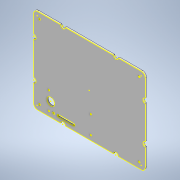
# Autodesk Inventor part: AcrylicCover
Saved by Autodesk Inventor 2022 (Build 260153000, 153)
## iProperties
Created: 2021-11-11
Part Number: AcrylicCover
Material: Generic
Document SubType Name: Modeling
Designer: Viktor
Density: 1 g/cm^3
Appearance: Default
Author: Viktor
Autodesk Inventor part; units mm, degrees
ref_plane "YZ Plane" through (0, 0, 0) normal (1, 0, 0) x (0, 1, 0)
ref_plane "XZ Plane" through (0, 0, 0) normal (0, 1, 0) x (-1, 0, 0)
ref_plane "XY Plane" through (0, 0, 0) normal (0, 0, 1) x (1, 0, 0)
sketch "Sketch1" plane through (0, 0, 0) normal (0, 0, 1) x (1, 0, 0)
  line L0 (-117, -89.5) -> (117, -89.5)
  line L1 (117, -89.5) -> (117, 89.5)
  line L2 (117, 89.5) -> (-117, 89.5)
  line L3 (-117, 89.5) -> (-117, -89.5)
  line L4 (-117, -89.5) -> (117, 89.5) construction
  line L5 (117, -89.5) -> (-117, 89.5) construction
  point P0 (0, 0)
  dimension "d0" = 234
  dimension "d1" = 179
  constraints: 12 end point, 2 midpoint, 2 parallel, 1 horizontal, 1 perpendicular
  measures "d0" distance between parallel lines of L1 L3
  measures "d1" distance between parallel lines of L0 L2
extrude "Extrusion1" add sketch "Sketch1" along normal blind 3
fillet "Fillet1" radius 8 4 edges at (117, -89.5, 1.5) (-117, -89.5, 1.5) (-117, 89.5, 1.5) (117, 89.5, 1.5)
sketch "Sketch2" plane through (0, 0, 3) normal (0, 0, 1) x (1, 0, 0)
  line L0 (-109, -89.5) -> (109, -89.5) construction
  arc A0 (-117, -81.5) -> (-109, -89.5) centre (-109, -81.5) ccw projected
  line L1 (-117, 81.5) -> (-117, -81.5) projected
  arc A1 (-109, 89.5) -> (-117, 81.5) centre (-109, 81.5) ccw projected
  line L2 (109, 89.5) -> (-109, 89.5) projected
  arc A2 (117, 81.5) -> (109, 89.5) centre (109, 81.5) ccw projected
  line L3 (117, -81.5) -> (117, 81.5) construction
  arc A3 (109, -89.5) -> (117, -81.5) centre (109, -81.5) ccw construction
  line L4 (-109, -89.5) -> (109, -89.5) projected
  circle A4 centre (55.5, -89.5) radius 5
  line L5 (117, -81.5) -> (117, 81.5) projected
  circle A5 centre (117, -39.5) radius 5
  line L6 (-170.275, 0) -> (170.275, 0) projected
  line L7 (0, 131.775) -> (0, -131.775) projected
  arc A6 (-117, -81.5) -> (-109, -89.5) centre (-109, -81.5) ccw construction
  circle A7 centre (-55.5, -89.5) radius 5
  circle A8 centre (-117, -39.5) radius 5
  line L8 (-109, 89.5) -> (109, 89.5) construction
  arc A9 (-109, 89.5) -> (-117, 81.5) centre (-109, 81.5) ccw
  arc A10 (117, 81.5) -> (109, 89.5) centre (109, 81.5) ccw construction
  line L9 (-109, 89.5) -> (109, 89.5)
  circle A11 centre (55.5, 89.5) radius 5
  circle A12 centre (117, 39.5) radius 5
  circle A13 centre (-117, 39.5) radius 5
  arc A14 (-109, 89.5) -> (-117, 81.5) centre (-109, 81.5) ccw construction
  circle A15 centre (-55.5, 89.5) radius 5
  point P0 (0, 0)
  point P1 (-50.5, -89.5)
  point P2 (-60.5, -89.5)
  point P3 (-117, -34.5)
  point P4 (-117, -44.5)
  point P5 (-117, 44.5)
  point P6 (-117, 34.5)
  point P7 (-60.5, 89.5)
  point P8 (-50.5, 89.5)
  point P9 (50.5, 89.5)
  point P10 (60.5, 89.5)
  point P11 (117, 44.5)
  point P12 (117, 34.5)
  point P13 (117, -34.5)
  point P14 (117, -44.5)
  point P15 (60.5, -89.5)
  point P16 (50.5, -89.5)
  dimension "d5" = 10
  dimension "d6" = 10
  dimension "d7" = 61.5
  dimension "d8" = 50
  constraints: 12 centre point, 10 symmetric about line, 8 point on circle, 4 end point, 3 point on line, 10 other
  measures "d5" diameter of A4
  measures "d6" diameter of A5
  measures "d7" distance from line of L3 A4.centre
  measures "d8" distance from line of L0 A5.centre
extrude "Extrusion2" cut sketch "Sketch2" against normal through all contours L5 A5 | A4 L4 | L1 A8 | A7 L4 | L1 A13 | A12 L5 | L2 A11 | A15 L2 picked at (116.6011, -41.1182) picked at (57.1182, -89.1011) picked at (-115.906, -37.9566) picked at (-53.8818, -89.1011) picked at (-115.906, 41.0434) picked at (115.4959, 40.7959) picked at (57.0242, 88.3266) picked at (-53.9758, 88.3266)
sketch "Sketch3" plane through (0, 0, 3) normal (0, 0, 1) x (1, 0, 0)
  circle A0 centre (104.5, -77.5) radius 1.75
  line L0 (117, -34.5) -> (117, 34.5) projected
  line L1 (60.5, -89.5) -> (109, -89.5) construction
  line L2 (0, 127.7397) -> (0, -127.7397) projected
  line L3 (-166.2397, 0) -> (166.2397, 0) projected
  circle A1 centre (-104.5, -77.5) radius 1.75
  circle A2 centre (104.5, 77.5) radius 1.75
  line L4 (60.5, 89.5) -> (109, 89.5) construction
  circle A3 centre (-104.5, 77.5) radius 1.75
  point P0 (0, 0)
  point P1 (-109, -89.5)
  point P2 (-109, 89.5)
  dimension "d11" = 3.5
  dimension "d33" = 209
  dimension "d34" = 155
  constraints: 7 symmetric about line, 4 centre point, 2 end point, 3 other
  measures "d11" diameter of A0
  measures "d33" distance of A1.centre A0.centre
  measures "d34" distance of A3.centre A1.centre
extrude "Extrusion3" cut sketch "Sketch3" against normal blind 10
sketch "Sketch4" plane through (0, 0, 3) normal (0, 0, 1) x (1, 0, 0)
  circle A0 centre (-81, -60.5) radius 8
  circle A1 centre (-75, -78.5) radius 2
  line L0 (-33, -78.5) -> (-65, -78.5) construction
  line L1 (-33, -76) -> (-65, -76)
  line L2 (-65, -81) -> (-33, -81)
  arc A2 (-33, -81) -> (-33, -76) centre (-33, -78.5) ccw
  arc A3 (-65, -76) -> (-65, -81) centre (-65, -78.5) ccw
  circle A4 centre (-85, -79.5) radius 1.5
  line L3 (-12.5, -60.5) -> (-95.5, -60.5) construction
  line L4 (-41, -83.5) -> (-41, -33.5) construction
  circle A5 centre (3, -79.5) radius 1.5
  circle A6 centre (-85, -41.5) radius 1.5
  circle A7 centre (3, -41.5) radius 1.5
  line L5 (-109, -89.5) -> (-60.5, -89.5) projected
  line L6 (-117, -44.5) -> (-117, -81.5) projected
  point P0 (0, 0)
  point P1 (-49, -78.5)
  dimension "d16" = 2.5
  dimension "d17" = 16
  dimension "d18" = 4
  dimension "d19" = 10
  dimension "d20" = 32
  dimension "d21" = 6
  dimension "d22" = 18
  dimension "d23" = 34
  dimension "d24" = 18
  dimension "d25" = 44
  dimension "d26" = 19
  dimension "d27" = 3
  dimension "d28" = 10
  dimension "d29" = 32
  dimension "d30" = 0
  constraints: 12 end point, 8 centre point, 4 point on circle, 4 tangent, 3 symmetric about line, 2 horizontal, 1 midpoint, 1 parallel, 1 vertical, 3 other
  measures "d16" radius of A3
  measures "d17" diameter of A0
  measures "d18" diameter of A1
  measures "d19" distance of L0.end A1.centre
  measures "d20" distance of L0.end L0.start
  measures "d21" horizontal distance of A0.centre A1.centre
  measures "d22" vertical distance of A1.centre A0.centre
  measures "d23" distance from line of L4 A1.centre
  measures "d24" distance from line of A1.centre L3
  measures "d25" distance from line of L4 A4.centre
  measures "d26" distance from line of L3 A4.centre
  measures "d27" diameter of A4
  measures "d28" distance from line of L5 A4.centre
  measures "d29" distance from line of L6 A4.centre
  measures "d30" vertical distance of A1.centre point (-49, -78.5)
extrude "Extrusion4" cut sketch "Sketch4" against normal through all
sketch "Sketch5" plane through (0, 0, 3) normal (0, 0, 1) x (1, 0, 0)
  circle A0 centre (-81, -60.5) radius 8 projected
  line L0 (-33, -81) -> (-65, -81) projected
  arc A1 (-65, -76) -> (-65, -81) centre (-65, -78.5) ccw projected
  line L1 (-65, -76) -> (-33, -76) projected
  arc A2 (-33, -81) -> (-33, -76) centre (-33, -78.5) ccw projected
  circle A3 centre (-85, -41.5) radius 1.5 projected
  circle A4 centre (3, -41.5) radius 1.5 projected
  circle A5 centre (-75, -78.5) radius 2 projected
  circle A6 centre (-85, -79.5) radius 1.5 projected
  circle A7 centre (3, -79.5) radius 1.5 projected
  circle A8 centre (-104.5, 77.5) radius 1.75 projected
  circle A9 centre (-104.5, -77.5) radius 1.75 projected
  circle A10 centre (104.5, 77.5) radius 1.75 projected
  circle A11 centre (104.5, -77.5) radius 1.75 projected
  arc A12 (117, 44.5) -> (117, 34.5) centre (117, 39.5) ccw projected
  line L2 (117, 44.5) -> (117, 81.5) projected
  arc A13 (117, 81.5) -> (109, 89.5) centre (109, 81.5) ccw projected
  line L3 (109, 89.5) -> (60.5, 89.5) projected
  arc A14 (50.5, 89.5) -> (60.5, 89.5) centre (55.5, 89.5) ccw projected
  line L4 (50.5, 89.5) -> (-50.5, 89.5) projected
  arc A15 (-60.5, 89.5) -> (-50.5, 89.5) centre (-55.5, 89.5) ccw projected
  line L5 (-60.5, 89.5) -> (-109, 89.5) projected
  arc A16 (-109, 89.5) -> (-117, 81.5) centre (-109, 81.5) ccw projected
  line L6 (-117, 81.5) -> (-117, 44.5) projected
  arc A17 (-117, 34.5) -> (-117, 44.5) centre (-117, 39.5) ccw projected
  line L7 (-117, 34.5) -> (-117, -34.5) projected
  arc A18 (-117, -44.5) -> (-117, -34.5) centre (-117, -39.5) ccw projected
  line L8 (-117, -44.5) -> (-117, -81.5) projected
  arc A19 (-117, -81.5) -> (-109, -89.5) centre (-109, -81.5) ccw projected
  line L9 (-109, -89.5) -> (-60.5, -89.5) projected
  arc A20 (-50.5, -89.5) -> (-60.5, -89.5) centre (-55.5, -89.5) ccw projected
  line L10 (-50.5, -89.5) -> (50.5, -89.5) projected
  arc A21 (60.5, -89.5) -> (50.5, -89.5) centre (55.5, -89.5) ccw projected
  line L11 (60.5, -89.5) -> (109, -89.5) projected
  arc A22 (109, -89.5) -> (117, -81.5) centre (109, -81.5) ccw projected
  line L12 (117, -81.5) -> (117, -44.5) projected
  arc A23 (117, -34.5) -> (117, -44.5) centre (117, -39.5) ccw projected
  line L13 (117, -34.5) -> (117, 34.5) projected
  point P0 (0, 0)
equation "\"d6\" = d5"
body "Solid1"
